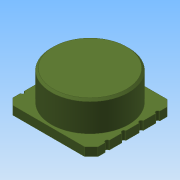
# Autodesk Inventor part: Drucksensor
Saved by Autodesk Inventor 2015 (Build 190159000, 159)
## iProperties
Created: 2015-07-10
Part Number: Drucksensor
Material: Stahl
Document SubType Name: Modeling
Designer: Johann
Density: 7.85 g/cm^3
Appearance: Olivgrün
Mass: 5 g
Surface Area: 1.33199 cm^2
Volume: 0.083813 cm^3
Author: Johann
Autodesk Inventor part; units mm, degrees
ref_plane "YZ Plane" through (0, 0, 0) normal (1, 0, 0) x (0, 1, 0)
ref_plane "XZ Plane" through (0, 0, 0) normal (0, 1, 0) x (-1, 0, 0)
ref_plane "XY Plane" through (0, 0, 0) normal (0, 0, 1) x (1, 0, 0)
sketch "Skizze1" plane through (0, 0, 0) normal (0, 0, 1) x (1, 0, 0)
  line L0 (-3.2, -3.1) -> (3.2, -3.1)
  line L1 (3.2, -3.1) -> (3.2, 3.1)
  line L2 (3.2, 3.1) -> (-3.2, 3.1)
  line L3 (-3.2, 3.1) -> (-3.2, -3.1)
  line L4 (-3.2, -3.1) -> (3.2, 3.1) construction
  line L5 (3.2, -3.1) -> (-3.2, 3.1) construction
  point P0 (0, 0)
  dimension "Breite_Keine_Pins" = 6.4
  dimension "Breite_Pins" = 6.2
  constraints: 12 end point, 2 midpoint, 2 parallel, 1 horizontal, 1 perpendicular
  measures "Breite_Keine_Pins" distance of L2.end L1.end
  measures "Breite_Pins" distance of L1.end L0.end
extrude "Extrusion1" add sketch "Skizze1" along normal blind 0.635
sketch "Skizze3" plane through (0, 0, 0.635) normal (0, 0, 1) x (1, 0, 0)
  line L0 (-3.2, -3.1) -> (3.2, -3.1) construction
  line L1 (3.2, -3.1) -> (3.2, 3.1) construction
  line L2 (3.2, 3.1) -> (-3.2, 3.1) construction
  line L3 (-3.2, 3.1) -> (-3.2, -3.1) construction
  line L4 (-3.2, 3.1) -> (-3.2, -3.1) construction
  arc A0 (-3.2, -2.05) -> (-3.2, -1.75) centre (-3.2, -1.9) ccw
  arc A1 (-3.2, -0.8) -> (-3.2, -0.5) centre (-3.2, -0.65) ccw
  arc A2 (-3.2, 1.75) -> (-3.2, 2.05) centre (-3.2, 1.9) ccw
  arc A3 (-3.2, 0.5) -> (-3.2, 0.8) centre (-3.2, 0.65) ccw
  line L5 (0, 3.1) -> (0, -3.1) construction
  line L6 (-3.2, -2.05) -> (-3.2, -1.75)
  line L7 (-3.2, -0.8) -> (-3.2, -0.5)
  line L8 (-3.2, 0.5) -> (-3.2, 0.8)
  line L9 (-3.2, 1.75) -> (-3.2, 2.05)
  arc A4 (3.2, -1.75) -> (3.2, -2.05) centre (3.2, -1.9) ccw
  arc A5 (3.2, -0.5) -> (3.2, -0.8) centre (3.2, -0.65) ccw
  arc A6 (3.2, 2.05) -> (3.2, 1.75) centre (3.2, 1.9) ccw
  arc A7 (3.2, 0.8) -> (3.2, 0.5) centre (3.2, 0.65) ccw
  line L10 (3.2, -2.05) -> (3.2, -1.75)
  line L11 (3.2, -0.8) -> (3.2, -0.5)
  line L12 (3.2, 0.5) -> (3.2, 0.8)
  line L13 (3.2, 1.75) -> (3.2, 2.05)
  point P0 (0, 0)
  dimension "d7" = 0.15
  dimension "d8" = 1.2
  dimension "d9" = 1.25
  dimension "d10" = 1.3
  dimension "d11" = 1.25
  constraints: 18 end point, 16 point on circle, 12 symmetric about line, 8 centre point, 4 collinear, 3 equal radius, 2 midpoint, 13 other
  measures "d7" radius of A0
  measures "d8" distance from line of A0.centre L0
  measures "d9" distance of A1.centre A0.centre
  measures "d10" distance of A3.centre A1.centre
  measures "d11" distance of A2.centre A3.centre
extrude "Extrusion3" cut sketch "Skizze3" against normal through all
sketch "Skizze2" plane through (0, 0, 0.635) normal (0, 0, 1) x (1, 0, 0)
  circle A0 centre (0, 0) radius 2.9
  dimension "Durchmesser_Sensor" = 5.8
  constraints: 1 centre point, 1 coincident
  measures "Durchmesser_Sensor" diameter of A0
extrude "Extrusion2" add sketch "Skizze2" along normal blind 2.245
sketch "Skizze5" plane through (0, 0, 0) normal (0, 0, -1) x (-1, 0, 0)
  line L0 (-2.8178, -1.6672) -> (-2.4426, -1.6672) construction
  line L1 (-2.4426, -1.6672) -> (-2.4426, -2.1689) construction
  line L2 (-2.4426, -2.1689) -> (-2.8178, -2.1689) construction
  line L3 (-2.8178, -2.1689) -> (-2.8178, -1.6672) construction
  line L4 (-3.2, -3.1) -> (-3.2, -2.05) projected
  line L5 (3.2, -3.1) -> (-3.2, -3.1) projected
  point P0 (0, 0)
  dimension "d14" = 0.3822
  dimension "d15" = 0.9311
  dimension "d16" = 0.3752
  dimension "d17" = 0.5016
  constraints: 2 other
  measures "d14" distance between parallel lines of L4 L3
  measures "d15" distance between parallel lines of L5 L2
  measures "d16" distance between parallel lines of L3 L1
  measures "d17" distance between parallel lines of L2 L0
chamfer "Fase1" distance 0.5 angle 45 4 edges at (3.2, 3.1, 0.3175) (3.2, -3.1, 0.3175) (-3.2, -3.1, 0.3175) (-3.2, 3.1, 0.3175)
chamfer "Fase2" distance 0.15 angle 45 1 edges at (-2.9, 0, 2.88)
fillet "Rundung1" radius 0.001 74 edges at (2.7, -3.1, 0.3175) (3.2, -2.6, 0.3175) (2.95, -2.85, 0.635) (0, -3.1, 0.635) (3.2, -2.325, 0.635) (3.2, -1.75, 0.3175) (3.2, -2.05, 0.3175) (3.2, -2.325, 0) (2.95, -2.85, 0) (0, -3.1, 0) (3.05, -1.9, 0.635) (3.05, -1.9, 0) (3.2, -1.275, 0) (3.2, -1.275, 0.635) (3.2, -0.5, 0.3175) (3.2, -0.8, 0.3175) (3.05, -0.65, 0.635) (3.05, -0.65, 0) (3.2, 0, 0.635) (3.2, 0.8, 0.3175) (3.2, 0.5, 0.3175) (3.2, 0, 0) (3.05, 0.65, 0.635) (3.05, 0.65, 0) (-2.9, 0, 0.635) (3.05, 1.9, 0.635) (3.2, 1.275, 0.635) (3.2, 2.05, 0.3175) (3.2, 1.75, 0.3175) (3.2, 1.275, 0) (3.05, 1.9, 0) (3.2, 2.325, 0) (3.2, 2.325, 0.635) (2.95, 2.85, 0.635) (3.2, 2.6, 0.3175) (2.7, 3.1, 0.3175) (2.95, 2.85, 0) (-2.9, 0, 2.73) (-2.75, 0, 2.88) (0, 3.1, 0.635) (0, 3.1, 0) (-2.95, -2.85, 0.635) (-2.7, -3.1, 0.3175) (-2.95, -2.85, 0) (-3.2, -2.6, 0.3175) (-3.2, -1.75, 0.3175) (-3.2, -2.05, 0.3175) (-3.2, -2.325, 0.635) (-3.05, -1.9, 0.635) (-3.2, -1.275, 0.635) (-3.05, -1.9, 0) (-3.2, -1.275, 0) (-3.2, -0.5, 0.3175) (-3.2, -0.8, 0.3175) (-3.05, -0.65, 0.635) (-3.05, -0.65, 0) (-3.2, 0, 0) (-3.2, 0, 0.635) (-3.05, 0.65, 0.635) (-3.2, 0.8, 0.3175) (-3.2, 0.5, 0.3175) (-3.05, 0.65, 0) (-3.2, 1.275, 0) (-3.2, 1.275, 0.635) (-3.05, 1.9, 0.635) (-3.2, 2.05, 0.3175) (-3.2, 1.75, 0.3175) (-3.05, 1.9, 0) (-3.2, 2.325, 0) (-3.2, 2.325, 0.635) (-2.95, 2.85, 0.635) (-2.95, 2.85, 0) (-2.7, 3.1, 0.3175) (-3.2, 2.6, 0.3175)
